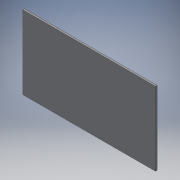
# Autodesk Inventor part: perfboard
Saved by Autodesk Inventor 2019 (Build 230136000, 136)
## iProperties
Created: 2021-03-14
Part Number: perfboard
Material: Generic
Document SubType Name: Modeling
Designer: Vijay
Density: 1 g/cm^3
Appearance: Default
Author: Vijay
Autodesk Inventor part; units mm, degrees
ref_plane "YZ Plane" through (0, 0, 0) normal (1, 0, 0) x (0, 1, 0)
ref_plane "XZ Plane" through (0, 0, 0) normal (0, 1, 0) x (-1, 0, 0)
ref_plane "XY Plane" through (0, 0, 0) normal (0, 0, 1) x (1, 0, 0)
sketch "Sketch1" plane through (0, 0, 0) normal (0, 0, 1) x (1, 0, 0)
  line L0 (-7.5335, 24.7663) -> (120.9955, 24.7663)
  line L1 (120.9955, 24.7663) -> (120.9955, -43.5803)
  line L2 (120.9955, -43.5803) -> (-7.5335, -43.5803)
  line L3 (-7.5335, -43.5803) -> (-7.5335, 24.7663)
  point P0 (0, 0)
  constraints: 8 end point, 2 parallel, 1 horizontal, 1 perpendicular
extrude "Extrusion1" add sketch "Sketch1" along normal blind 1.64
fillet "Fillet1" radius 10 4 edges at (120.9955, 24.7663, 0.82) (120.9955, -43.5803, 0.82) (-7.5335, 24.7663, 0.82) (-7.5335, -43.5803, 0.82)
body "Solid1"
